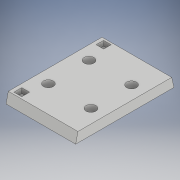
# Autodesk Inventor part: BottomHolderThrustMotorHousing
Saved by Autodesk Inventor 2019 (Build 230136000, 136)
## iProperties
Created: 2018-09-19
Part Number: BottomHolderThrustMotorHousing
Material: Generic
Document SubType Name: Modeling
Designer: hale985
Density: 1 g/cm^3
Appearance: Default
Author: hale985
Autodesk Inventor part; units mm, degrees
sketch "Sketch1" plane through (0, 0, 0) normal (1, 0, 0) x (0, 1, 0)
  circle A0 centre (0, 0) radius 3.937
  circle A1 centre (0, 0) radius 7.747
  dimension "d0" = 7.874
  dimension "d1" = 3.81
  constraints: 2 centre point, 1 coincident
  measures "d0" diameter of A0
  measures "d1" radial gap between concentric circles of A0 A1
ref_plane "Work Plane2" through (0, 0, 0) normal (-1, 0, 0) x (0, 0, 1)
sketch "Sketch2" plane through (0, 0, 0) normal (-1, 0, 0) x (0, 0, 1)
  circle A0 centre (0, 0) radius 7.7384
  circle A1 centre (0, 0) radius 7.747
  constraints: 2 centre point, 2 coincident
ref_plane "Work Plane4" through (-2.54, 0, 0) normal (-1, 0, 0) x (0, 0, 1)
sketch "Sketch3" plane through (-2.54, 0, 0) normal (-1, 0, 0) x (0, 0, 1)
  line L0 (19.05, 48.5955) -> (-19.05, 48.5955)
  circle A0 centre (0, 0) radius 7.747 projected
  line L1 (7.747, 0) -> (19.05, 48.5955)
  line L2 (-7.747, 0) -> (-19.05, 48.5955)
  arc A1 (7.747, 0) -> (-7.747, 0) centre (0, 0) ccw
  line L3 (-14.2521, 44.7855) -> (14.2521, 44.7855)
  line L4 (14.2521, 44.7855) -> (6.1161, 9.806)
  arc A2 (6.1161, 9.806) -> (-6.1161, 9.806) centre (0, 0) ccw
  line L5 (-6.1161, 9.806) -> (-14.2521, 44.7855)
  dimension "d6" = 38.1
  dimension "d7" = 19.05
  dimension "d8" = 3.81
  constraints: 12 end point, 6 point on circle, 2 centre point, 1 concentric, 1 horizontal, 3 other
  measures "d6" distance of L0.start L0.end
  measures "d7" horizontal distance of L0.start point (0, 0)
  measures "d8" distance between parallel lines of L0 L3
ref_plane "Work Plane5" through (3.81, 0, 0) normal (1, 0, 0) x (0, 0, -1)
sketch "Sketch4" plane through (3.81, 0, 0) normal (1, 0, 0) x (0, 0, -1)
  line L0 (14.2521, 44.7855) -> (6.1161, 9.806) projected
  line L1 (14.2521, 44.7855) -> (6.1161, 9.806) projected
  arc A0 (6.1161, 9.806) -> (-6.1161, 9.806) centre (0, 0) ccw projected
  line L2 (-6.1161, 9.806) -> (-14.2521, 44.7855) projected
  line L3 (-14.2521, 44.7855) -> (14.2521, 44.7855) projected
  line L4 (19.05, 48.5955) -> (-19.05, 48.5955) projected
  line L5 (-19.05, 48.5955) -> (-7.747, 0) projected
  line L6 (7.747, 0) -> (19.05, 48.5955) projected
  line L7 (-14.2521, 44.7855) -> (14.2521, 44.7855) projected
  line L8 (14.2521, 44.7855) -> (18.1638, 44.7855)
  line L9 (14.2521, 44.7855) -> (-14.2521, 44.7855)
  line L10 (-14.2521, 44.7855) -> (-18.1638, 44.7855)
  line L11 (-19.05, 48.5955) -> (-7.747, 0) projected
  line L12 (-19.05, 48.5955) -> (-18.1638, 44.7855)
  line L13 (18.1638, 44.7855) -> (19.05, 48.5955)
  line L14 (-19.05, 48.5955) -> (19.05, 48.5955) projected
  line L15 (19.05, 48.5955) -> (-19.05, 48.5955)
  line L16 (18.1638, 44.7855) -> (-18.1638, 44.7855)
  arc A1 (7.747, 0) -> (-7.747, 0) centre (0, 0) ccw projected
  constraints: 14 end point, 5 point on line, 4 collinear, 1 horizontal
extrude "Extrusion4" add sketch "Sketch4" along normal blind 20.6375 contours L3 L10 L5 L4 L6 L8
ref_plane "Work Plane7" through (-2.54, 44.7855, -14.2521) normal (0, -1, 0) x (1, 0, 0)
ref_plane "Work Plane6" through (-2.54, 44.7855, -14.2521) normal (0, -1, 0) x (1, 0, 0)
sketch "Sketch6" plane through (-2.54, 44.7855, -14.2521) normal (0, -1, 0) x (1, 0, 0)
  line L0 (6.35, 32.4159) -> (26.9875, 32.4159) projected
  line L1 (13.4874, 32.4159) -> (13.4874, 26.0989)
  line L2 (26.9875, 32.4159) -> (26.9875, -3.9117) projected
  point P0 (2.54, 14.2521)
  dimension "d20" = 13.5001
  constraints: 2 end point, 1 point on line, 1 vertical
  measures "d20" distance between parallel lines of L2 L1
ref_plane "Work Plane1" through (10.9347, 0, 0) normal (1, 0, 0) x (0, 0, -1)
ref_plane "Work Plane3" through (0, 0, 0) normal (1, 0, 0) x (0, 0, -1)
sketch "Sketch10" plane through (0, 0, 0) normal (1, 0, 0) x (0, 0, -1)
  circle A0 centre (0, 0) radius 1.4542
  constraints: 1 centre point, 1 coincident
extrude "Extrusion7" cut sketch "Sketch10" against normal blind 22.225
sketch "Sketch12" plane through (3.81, 0, 0) normal (-1, 0, 0) x (0, 0, 1)
  line L0 (18.1638, 44.7855) -> (-18.1638, 44.7855) projected
  line L1 (19.05, 48.5955) -> (18.1638, 44.7855) projected
  line L2 (-19.05, 48.5955) -> (19.05, 48.5955) projected
  line L3 (-19.05, 48.5955) -> (19.05, 48.5955) projected
  line L4 (18.1638, 44.7855) -> (-18.1638, 44.7855) projected
  line L5 (-19.05, 48.5955) -> (19.05, 48.5955) projected
  line L6 (-18.1638, 44.7855) -> (-19.05, 48.5955) projected
  line L7 (18.1638, 44.7855) -> (-18.1638, 44.7855) projected
  line L8 (-19.05, 48.5955) -> (19.05, 48.5955) projected
  line L9 (19.05, 48.5955) -> (-19.05, 48.5955)
  line L10 (-9.4207, 44.7855) -> (-18.1638, 44.7855) projected
  line L11 (-19.05, 48.5955) -> (-18.1638, 44.7855)
  line L12 (18.1638, 44.7855) -> (-18.1638, 44.7855) projected
  line L13 (-18.1638, 44.7855) -> (18.1638, 44.7855)
  line L14 (18.1638, 44.7855) -> (19.05, 48.5955)
  line L15 (19.05, 48.5955) -> (18.1638, 44.7855) projected
  line L16 (19.05, 48.5955) -> (18.1638, 44.7855) projected
  line L17 (-18.1638, 44.7855) -> (-19.05, 48.5955) projected
  line L18 (-18.1638, 44.7855) -> (-19.05, 48.5955) projected
  point P0 (0, 0)
  point P1 (9.4207, 48.5955)
  point P2 (9.4207, 44.7855)
  point P3 (6.3245, 44.7855)
  point P4 (6.3245, 48.5955)
  point P5 (-6.3245, 48.5955)
  point P6 (-6.3245, 44.7855)
  point P7 (-9.4207, 48.5955)
  constraints: 8 end point, 2 collinear, 1 parallel
extrude "Extrusion8" add sketch "Sketch12" along normal blind 6.35
sketch "Sketch13" plane through (24.4475, 44.7855, -18.1638) normal (0, -1, 0) x (1, 0, 0)
  line L0 (-26.9875, 0) -> (-26.9875, 36.3276) projected
  line L1 (0, 36.3276) -> (0, 0) projected
  line L2 (-26.9875, 36.3276) -> (0, 36.3276) projected
  line L3 (-26.9875, -0.8862) -> (0, -0.8862) projected
  line L4 (0, 37.2138) -> (-26.9875, 37.2138) projected
  point P0 (-24.4475, 18.1638)
  point P1 (-21.7476, 26.0364)
  point P2 (-21.7476, 10.2912)
  dimension "d35" = 21.7476
  dimension "d36" = 21.7476
  dimension "d38" = 11.1774
  dimension "d39" = 11.1774
  measures "d35" distance from line of L1 point (-21.748, 10.291)
  measures "d36" distance from line of L1 point (-21.748, 26.036)
  measures "d38" distance from line of L3 point (-21.748, 10.291)
  measures "d39" distance from line of L4 point (-21.748, 26.036)
ref_plane "Work Plane8" through (10.9537, 0, 0) normal (1, 0, 0) x (0, 0, -1)
hole "Hole2" at (2.6999, 44.7855, -7.8726) at (2.6999, 44.7855, 7.8726) direction (0, 1, 0) diameter 3.81 end through all
mirror "Mirror2" about plane through (10.9537, 0, 0) normal (1, 0, 0) of "Hole2"
sketch "Sketch14" plane through (24.4475, 44.7855, -18.1638) normal (0, -1, 0) x (1, 0, 0)
  line L0 (-25.5905, 0.7648) -> (-22.5425, 0.7648)
  line L1 (-22.5425, 0.7648) -> (-22.5425, 3.8128)
  line L2 (-22.5425, 3.8128) -> (-25.5905, 3.8128)
  line L3 (-25.5905, 3.8128) -> (-25.5905, 0.7648)
  line L4 (-26.9875, -0.8862) -> (0, -0.8862) projected
  line L5 (-26.9875, 0) -> (-26.9875, 36.3276) projected
  line L6 (-25.5905, 32.6418) -> (-22.6695, 32.6418)
  line L7 (-22.6695, 32.6418) -> (-22.6695, 35.5628)
  line L8 (-22.6695, 35.5628) -> (-25.5905, 35.5628)
  line L9 (-25.5905, 35.5628) -> (-25.5905, 32.6418)
  line L10 (0, 37.2138) -> (-26.9875, 37.2138) projected
  point P0 (-24.4475, 18.1638)
  dimension "d47" = 3.048
  dimension "d48" = 3.048
  dimension "d49" = 1.651
  dimension "d50" = 1.397
  dimension "d51" = 2.921
  dimension "d52" = 2.921
  dimension "d53" = 1.651
  dimension "d54" = 1.397
  constraints: 16 end point, 4 parallel, 2 horizontal, 2 perpendicular
  measures "d47" distance of L2.end L1.end
  measures "d48" distance of L1.end L0.end
  measures "d49" distance between parallel lines of L4 L0
  measures "d50" distance between parallel lines of L5 L3
  measures "d51" distance of L8.end L7.end
  measures "d52" distance of L7.end L6.end
  measures "d53" distance between parallel lines of L10 L8
  measures "d54" distance between parallel lines of L5 L9
extrude "Extrusion9" cut sketch "Sketch14" against normal blind 1.905
body "Solid1"
